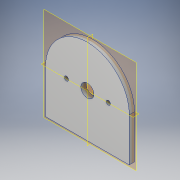
# Autodesk Inventor part: Boom Hinge
Saved by Autodesk Inventor 2019 (Build 230136000, 136)
## iProperties
Created: 2018-10-28
Part Number: Boom Hinge
Material: Aluminum 6061
Document SubType Name: Modeling
Designer: Alex Barnett
Density: 2.7 g/cm^3
Appearance: Aluminum - Flat
Mass: 186.738 g
Surface Area: 249.498 cm^2
Volume: 69.1622 cm^3
Author: Alex Barnett
Autodesk Inventor part; units mm, degrees
sketch "Sketch1" plane through (0, 0, 0) normal (0, 0, 1) x (1, 0, 0)
  arc A0 (50.8, 0) -> (-50.8, 0) centre (0, 0) ccw
  line L0 (50.8, 0) -> (50.8, -52.7558)
  line L1 (50.8, -52.7558) -> (-50.8, -52.7558)
  line L2 (-50.8, -52.7558) -> (-50.8, 0)
  line L3 (0, 71.5112) -> (0, -73.467) projected
  dimension "d2" = 52.7558
  dimension "d3" = 50.8
  dimension "d22" = 0
  constraints: 6 end point, 2 point on circle, 1 centre point, 1 parallel
  measures "d2" distance of L0.start L0.end
  measures "d3" radius of A0
  measures "d22" distance from line of L3 A0.centre
extrude "Extrusion1" add sketch "Sketch1" along normal mid plane 6.35
sketch "Sketch2" plane through (0, 0, 3.175) normal (0, 0, 1) x (1, 0, 0)
  point P0 (0, 0)
  point P1 (0, 0)
  constraints: 1 coincident
hole "Hole1" at (0, 0, 3.175) direction (0, 0, -1) diameter 15.875 end through all
sketch "Sketch5" plane through (0, 0, 3.175) normal (0, 0, 1) x (1, 0, 0)
  circle A0 centre (-25.4, 0) radius 2.54
  line L0 (0, 50.8056) -> (0, 0) construction
  circle A1 centre (25.4, 0) radius 2.54
  dimension "d31" = 5.08
  dimension "d32" = 25.4
  constraints: 2 centre point, 2 end point, 1 symmetric about line, 1 vertical, 1 other
  measures "d31" diameter of A0
  measures "d32" distance of L0.end A0.centre
hole "Hole4" at (-25.4, 0, 3.175) at (25.4, 0, 3.175) direction (0, 0, -1) diameter 5.08 end through all
body "Solid1"
